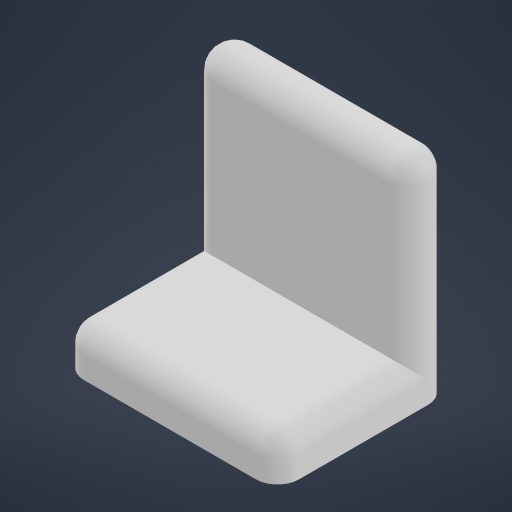
# Autodesk Inventor part: Marker Holder 90 deg
Saved by Autodesk Inventor 2024.1 (Build 281209000, 209)
## iProperties
Created: 2023-09-09
Part Number: Marker Holder 90 deg
Material: Generic
Document SubType Name: Modeling
Designer: User
Density: 1 g/cm^3
Appearance: Default
Author: User
Autodesk Inventor part; units mm, degrees
ref_plane "YZ Plane" through (0, 0, 0) normal (1, 0, 0) x (0, 1, 0)
ref_plane "XZ Plane" through (0, 0, 0) normal (0, 1, 0) x (-1, 0, 0)
ref_plane "XY Plane" through (0, 0, 0) normal (0, 0, 1) x (1, 0, 0)
sketch "Sketch1" plane through (0, 0, 0) normal (0, 0, 1) x (1, 0, 0)
  line L0 (0, 0) -> (-50, 0)
  line L1 (-50, 0) -> (-50, 50)
  line L2 (-50, 50) -> (0, 50)
  line L3 (0, 50) -> (0, 0)
  dimension "d0" = 50
  dimension "d1" = 50
  constraints: 8 end point, 2 parallel, 1 horizontal, 1 perpendicular
  measures "d0" distance of L1.end L2.end
  measures "d1" distance of L0.end L1.end
extrude "Extrusion1" add sketch "Sketch1" along normal blind 10
sketch "Sketch2" plane through (0, 0, 10) normal (0, 0, 1) x (1, 0, 0)
  line L0 (-49.9965, 0) -> (0.0035, 0)
  line L1 (0.0035, 0) -> (0.0035, 10)
  line L2 (0.0035, 10) -> (-49.9965, 10)
  line L3 (-49.9965, 10) -> (-49.9965, 0)
  point P0 (0, 0)
  dimension "d4" = 50
  dimension "d5" = 10
  constraints: 8 end point, 2 parallel, 1 horizontal, 1 perpendicular
  measures "d4" distance of L2.end L1.end
  measures "d5" distance of L1.end L0.end
extrude "Extrusion2" add sketch "Sketch2" along normal blind 30
fillet "Fillet3" radius 5 6 edges at (-49.9965, 10, 25) (0.0035, 10, 25) (0, 30, 10) (-50, 25, 10) (-50, 25, 0) (0, 25, 0)
fillet "Fillet5" radius 5 11 edges at (-1.4609, 8.5355, 40) (-24.9965, 10, 40) (-48.532, 8.5355, 40) (-49.9965, 2.5, 40) (0.0035, 2.5, 40) (-1.4644, 50, 8.5356) (-48.5356, 50, 8.5356) (-1.4645, 50, 1.4645) (-48.5355, 50, 1.4645) (-25, 50, 0) (-25, 50, 10)
body "Solid1"
